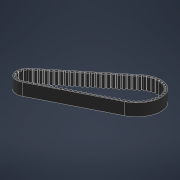
# Autodesk Inventor part: Parametric HTD Belt v1
Saved by Autodesk Inventor 2021 (Build 250183000, 183)
## iProperties
Created: 2020-06-05
Part Number: Parametric HTD Belt v1
Material: Rubber
Document SubType Name: Modeling
Designer: Bryce
Density: 0.93 g/cm^3
Appearance: Rubber - Black
Author: Bryce
Autodesk Inventor part; units mm, degrees
ref_plane "YZ Plane" through (0, 0, 0) normal (1, 0, 0) x (0, 1, 0)
ref_plane "XY Plane" through (0, 0, 0) normal (0, 0, 1) x (1, 0, 0)
sketch "top teeth placement" plane through (0, 0, 0) normal (0, 1, 0) x (-1, 0, 0)
  arc A0 (1.9259, -14.1939) -> (1.9259, 14.1939) centre (0, 0) ccw construction
  line L0 (1.9259, -14.1939) -> (-102.6854, -28.3878) construction
  line L1 (1.9259, 14.1939) -> (-102.6854, 28.3878) construction
  arc A1 (-102.6854, 28.3878) -> (-102.6854, -28.3878) centre (-106.5371, 0) ccw construction
  arc A2 (1.9259, -14.1939) -> (6.6643, -12.6792) centre (0, 0) ccw construction
  arc A3 (-107.1039, -28.6423) -> (-102.6854, -28.3878) centre (-106.5371, 0) ccw construction
  arc A4 (-112.0689, -28.1087) -> (-107.1039, -28.6423) centre (-106.5371, 0) ccw construction
  line L2 (1.9259, -14.1939) -> (0, 0) construction
  line L3 (0, 0) -> (6.6643, -12.6792) construction
  line L4 (-107.1039, -28.6423) -> (-106.5371, 0) construction
  line L5 (-106.5371, 0) -> (-112.0689, -28.1087) construction
  point P0 (-3.0287, -14.8661)
  point P1 (-7.9833, -15.5384)
  point P2 (-12.9379, -16.2106)
  point P3 (-17.8925, -16.8829)
  point P4 (-22.8471, -17.5551)
  point P5 (-27.8018, -18.2274)
  point P6 (-1.9025, 14.7133)
  point P7 (-6.8571, 15.3856)
  point P8 (-32.7564, -18.8996)
  point P9 (-37.711, -19.5719)
  point P10 (-42.6656, -20.2442)
  point P11 (-47.6202, -20.9164)
  point P12 (-52.5748, -21.5887)
  point P13 (-57.5294, -22.2609)
  point P14 (-62.484, -22.9332)
  point P15 (-67.4386, -23.6054)
  point P16 (-72.3932, -24.2777)
  point P17 (-77.3478, -24.9499)
  point P18 (-82.3024, -25.6222)
  point P19 (-87.257, -26.2944)
  point P20 (-92.2116, -26.9667)
  point P21 (-97.1662, -27.6389)
  point P22 (-102.1208, -28.3112)
  dimension "pitch" = 5
  dimension "r_d35" = 105
  dimension "r_d36" = 40
  dimension "d17" = 28.6479
  dimension "d18" = 57.2958
  dimension "d30" = 5
  dimension "d35" = 105.5697
  dimension "d36" = 41.1366
  dimension "d39" = 20
  dimension "d41" = 5
  dimension "d44" = 4.4303
  dimension "d45" = 97.7268
  dimension "d48" = 10
  dimension "d50" = 5
  dimension "d52" = 3.8634
  dimension "d62" = 5
  dimension "d71" = 106.5371
  constraints: 12 end point, 11 point on circle, 5 centre point, 4 coincident, 4 tangent, 3 concentric, 1 horizontal alignment, 1 point on line, 28 other
  measures "d17" diameter of A0
  measures "d18" diameter of A1
  measures "d30" distance of L2.start point (-3.029, -14.866)
  measures "d35" distance of L0.start L0.end
  measures "d52" distance of point (-1.902, 14.713) L1.start
  measures "d62" distance of point (-1.902, 14.713) point (-6.857, 15.386)
  measures "d71" distance of A1.centre point (0, 0)
sketch "htd profile" plane through (0, 0, 0) normal (0, 1, 0) x (-1, 0, 0)
  line L0 (-107.1039, -28.6423) -> (-106.5371, 0) construction
  arc A0 (-102.6854, 28.3878) -> (-102.6854, -28.3878) centre (-106.5371, 0) ccw construction
  arc A1 (3.2344, -12.9293) -> (0.3276, -13.3237) centre (1.7458, -12.8665) ccw
  line L1 (1.9259, -14.1939) -> (-102.6854, -28.3878) construction
  arc A2 (-0.0238, -13.8817) -> (0.3276, -13.3237) centre (-0.0816, -13.4556) ccw
  arc A3 (3.2344, -12.9293) -> (3.7219, -13.3735) centre (3.664, -12.9474) ccw
  line L2 (1.5454, -11.39) -> (1.8224, -13.4313) construction
  line L3 (4.3263, -13.2915) -> (3.7219, -13.3735)
  line L4 (-0.0238, -13.8817) -> (-0.6283, -13.9637)
  line L5 (4.4933, -14.5221) -> (-0.4613, -15.1943)
  line L6 (4.4933, -14.5221) -> (4.3263, -13.2915)
  line L7 (-0.4613, -15.1943) -> (-0.6283, -13.9637)
  line L8 (1.7458, -12.8665) -> (2.016, -14.8582) construction
  arc A4 (-105.6161, -27.5943) -> (-108.549, -27.5363) centre (-107.0774, -27.303) ccw
  arc A5 (-108.9822, -28.0335) -> (-108.549, -27.5363) centre (-108.9737, -27.6036) ccw
  arc A6 (-105.6161, -27.5943) -> (-105.2029, -28.1083) centre (-105.1944, -27.6784) ccw
  line L9 (-107.0479, -25.8133) -> (-107.0886, -27.8729) construction
  line L10 (-104.593, -28.1204) -> (-105.2029, -28.1083)
  line L11 (-108.9822, -28.0335) -> (-109.5921, -28.0214)
  line L12 (-104.6176, -29.362) -> (-109.6166, -29.2631)
  line L13 (-104.6176, -29.362) -> (-104.593, -28.1204)
  line L14 (-109.6166, -29.2631) -> (-109.5921, -28.0214)
  line L15 (-107.0774, -27.303) -> (-107.1171, -29.3126) construction
  line L16 (-104.6044, -28.6917) -> (-109.6034, -28.5928) construction
  line L17 (1.9259, 14.1939) -> (-102.6854, 28.3878) construction
  arc A7 (-3.5007, 13.8431) -> (-0.5939, 13.4487) centre (-2.0826, 13.3859) ccw
  arc A8 (-0.1065, 13.8929) -> (-0.5939, 13.4487) centre (-0.1643, 13.4668) ccw
  arc A9 (-3.5007, 13.8431) -> (-3.8522, 14.4011) centre (-3.91, 13.975) ccw
  line L18 (-2.2829, 11.9094) -> (-2.006, 13.9507) construction
  line L19 (-4.4566, 14.4831) -> (-3.8522, 14.4011)
  line L20 (-0.1065, 13.8929) -> (0.498, 13.8109)
  line L21 (-4.2896, 15.7138) -> (0.665, 15.0415)
  line L22 (-4.2896, 15.7138) -> (-4.4566, 14.4831)
  line L23 (0.665, 15.0415) -> (0.498, 13.8109)
  line L24 (-2.0826, 13.3859) -> (-1.8123, 15.3777) construction
  point P0 (0, 0)
  point P1 (-1.9025, 14.7133)
  dimension "d93" = 1.49
  dimension "d94" = 0.43
  dimension "d95" = 2.06
  dimension "d97" = 3.5
  dimension "d98" = 5
  dimension "d99" = 0.5715
  dimension "d101" = 3.78
  dimension "d102" = 1.49
  dimension "d103" = 0.43
  dimension "d104" = 2.06
  dimension "d105" = 3.5
  dimension "d106" = 5
  dimension "d107" = 3.78
  dimension "d109" = 0.5715
  dimension "d150" = 1.49
  dimension "d151" = 0.43
  dimension "d152" = 2.06
  dimension "d153" = 3.5
  dimension "d154" = 5
  dimension "d155" = 3.78
  dimension "d157" = 0.5715
  constraints: 44 end point, 21 point on circle, 19 tangent, 12 perpendicular, 9 centre point, 8 point on line, 7 parallel, 3 collinear, 3 equal radius, 3 midpoint, 1 line through centre
  measures "d93" radius of A1
  measures "d94" radius of A2
  measures "d95" distance of L2.start L2.end
  measures "d97" distance from line of L5 L2.start
  measures "d98" distance between parallel lines of L7 L6
  measures "d99" distance between parallel lines of L1 L4
  measures "d101" distance of L4.start L3.end
  measures "d102" radius of A4
  measures "d103" radius of A5
  measures "d104" distance of L9.start L9.end
  measures "d105" distance from line of L12 L9.start
  measures "d106" distance between parallel lines of L14 L13
  measures "d107" distance of L11.start L10.end
  measures "d109" distance between parallel lines of L16 L10
  measures "d150" radius of A7
  measures "d151" radius of A8
  measures "d152" distance of L18.start L18.end
  measures "d153" distance from line of L21 L18.start
  measures "d154" distance between parallel lines of L23 L22
  measures "d155" distance of L20.start L19.end
  measures "d157" distance between parallel lines of L17 L19
extrude "Top/Left Base Tooth" add sketch "htd profile" against normal mid plane 15 contours A3 L3 L6 L5 L7 L4 A2 A1
pattern_sketch "Top Teeth" of "Top/Left Base Tooth" from (-1.9259, 0, -14.1939) copies at (3.0287, 0, -14.8661) at (7.9833, 0, -15.5384) at (12.9379, 0, -16.2106) at (17.8925, 0, -16.8829) at (22.8471, 0, -17.5551) at (27.8018, 0, -18.2274) at (32.7564, 0, -18.8996) at (37.711, 0, -19.5719) at (42.6656, 0, -20.2442) at (47.6202, 0, -20.9164) at (52.5748, 0, -21.5887) at (57.5294, 0, -22.2609) at (62.484, 0, -22.9332) at (67.4386, 0, -23.6054) at (72.3932, 0, -24.2777) at (77.3478, 0, -24.9499) at (82.3024, 0, -25.6222) at (87.257, 0, -26.2944) at (92.2116, 0, -26.9667) at (97.1662, 0, -27.6389) at (102.1208, 0, -28.3112)
pattern_circular "Left Teeth" count 8 over 160 about axis through (0, 0, 0) along (0, 1, 0) of "Top/Left Base Tooth"
extrude "Right Base Tooth" add sketch "htd profile" along normal mid plane 15 contours A6 L10 L13 L12 L14 L11 A5 A4
pattern_circular "Right Teeth" count 19 over 180 about axis through (106.5371, 0, 0) along (0, -1, 0) of "Right Base Tooth"
sketch "bottom teeth placement" plane through (0, 0, 0) normal (0, 1, 0) x (-1, 0, 0)
  arc A0 (1.9259, -14.1939) -> (1.9259, 14.1939) centre (0, 0) ccw construction
  line L0 (1.9259, -14.1939) -> (-102.6854, -28.3878) construction
  line L1 (1.9259, 14.1939) -> (-102.6854, 28.3878) construction
  arc A1 (-102.6854, 28.3878) -> (-102.6854, -28.3878) centre (-106.5371, 0) ccw construction
  point P0 (-1.9025, 14.7133)
  point P1 (-6.8571, 15.3856)
  point P2 (-11.8117, 16.0578)
  point P3 (-16.7663, 16.7301)
  point P4 (-21.7209, 17.4023)
  point P5 (-26.6755, 18.0746)
  point P6 (-31.6301, 18.7468)
  point P7 (-36.5847, 19.4191)
  point P8 (-41.5393, 20.0913)
  point P9 (-46.4939, 20.7636)
  point P10 (-51.4485, 21.4358)
  point P11 (-56.4031, 22.1081)
  point P12 (-61.3577, 22.7803)
  point P13 (-66.3123, 23.4526)
  point P14 (-71.2669, 24.1248)
  point P15 (-76.2215, 24.7971)
  point P16 (-81.1761, 25.4694)
  point P17 (-86.1307, 26.1416)
  point P18 (-91.0853, 26.8139)
  point P19 (-96.0399, 27.4861)
  point P20 (-100.9945, 28.1584)
  dimension "d144" = 5
  dimension "d147" = 40
  dimension "pitch" = 5
  dimension "d123" = 28.6479
  dimension "d124" = 57.2958
  dimension "d126" = 105.5697
  dimension "d127" = 41.1366
  dimension "d131" = 97.7268
  dimension "d134" = 3.8634
  dimension "d135" = 5
  dimension "d136" = 106.5371
  constraints: 4 end point, 4 point on circle, 4 tangent, 2 centre point, 2 coincident, 1 horizontal alignment, 1 point on line, 21 other
  measures "d123" diameter of A0
  measures "d124" diameter of A1
  measures "d126" distance of L0.start L0.end
  measures "d134" distance of point (-1.902, 14.713) L1.start
  measures "d135" distance of point (-1.902, 14.713) point (-6.857, 15.386)
  measures "d136" distance of A1.centre point (0, 0)
extrude "Bottom Base Tooth" add sketch "htd profile" along normal mid plane 15 contours A9 L19 L22 L21 L23 L20 A8 A7
pattern_sketch "Bottom Teeth" of "Bottom Base Tooth" from (1.9025, 0, 14.7133) copies at (6.8571, 0, 15.3856) at (11.8117, 0, 16.0578) at (16.7663, 0, 16.7301) at (21.7209, 0, 17.4023) at (26.6755, 0, 18.0746) at (31.6301, 0, 18.7468) at (36.5847, 0, 19.4191) at (41.5393, 0, 20.0913) at (46.4939, 0, 20.7636) at (51.4485, 0, 21.4358) at (56.4031, 0, 22.1081) at (61.3577, 0, 22.7803) at (66.3123, 0, 23.4526) at (71.2669, 0, 24.1248) at (76.2215, 0, 24.7971) at (81.1761, 0, 25.4694) at (86.1307, 0, 26.1416) at (91.0853, 0, 26.8139) at (96.0399, 0, 27.4861) at (100.9945, 0, 28.1584)
sketch "Sketch7" plane through (0, 0, 0) normal (0, 1, 0) x (-1, 0, 0)
  line L0 (1.9259, 14.1939) -> (-102.6854, 28.3878) construction
  arc A0 (1.9259, -14.1939) -> (1.9259, 14.1939) centre (0, 0) ccw construction
  line L1 (1.9259, -14.1939) -> (-102.6854, -28.3878) construction
  arc A1 (-102.6854, 28.3878) -> (-102.6854, -28.3878) centre (-106.5371, 0) ccw construction
  line L2 (1.849, 13.6276) -> (-102.7622, 27.8215)
  arc A2 (-102.7622, 27.8215) -> (-102.7622, -27.8215) centre (-106.5371, 0) ccw
  line L3 (-102.7622, -27.8215) -> (1.849, -13.6276)
  arc A3 (1.849, -13.6276) -> (1.849, 13.6276) centre (0, 0) ccw
  line L4 (-102.5549, -29.3494) -> (2.0563, -15.1555)
  arc A4 (2.0563, -15.1555) -> (2.0563, 15.1555) centre (0, 0) ccw
  line L5 (2.0563, 15.1555) -> (-102.5549, 29.3494)
  arc A5 (-102.5549, 29.3494) -> (-102.5549, -29.3494) centre (-106.5371, 0) ccw
  line L6 (-0.0238, -13.8817) -> (-1.2327, -14.0457) construction
  line L7 (-104.5079, -29.3116) -> (4.4933, -14.5221) construction
  arc A6 (3.2344, -12.9293) -> (0.3276, -13.3237) centre (1.7458, -12.8665) ccw construction
  arc A7 (3.2344, -12.9293) -> (0.3276, -13.3237) centre (1.7458, -12.8665) ccw construction
  line L8 (1.5454, -11.39) -> (1.849, -13.6276) construction
  dimension "d163" = 3.8
  constraints: 10 end point, 9 point on circle, 4 centre point, 2 point on line, 1 coincident, 1 collinear, 1 perpendicular, 6 other
  measures "d163" distance from line of L4 point (1.545, -11.39)
extrude "Belt" add sketch "Sketch7" along normal mid plane 15
equation "\"pitch\" = 5"
equation "\"r_d36\" = 40"
equation "\"d30\" = pitch"
equation "\"d41\" = pitch"
equation "\"d44\" = pitch + r_d35 - d35"
equation "\"d50\" = pitch"
equation "\"d62\" = pitch"
equation "\"d144\" = 5"
equation "\"d147\" = 40"
equation "\"r_d45\" = 95"
equation "\"pulley_1_angle\" = 20deg"
equation "\"pulley_2_angle\" = 10deg"
equation "\"d108\" = 5"
equation "\"d156\" = 5"
equation "\"center_distance\" = 106.53707"
equation "\"f_d35\" = 105"
equation "\"htd_pld\" = 0.5715"
equation "\"missing_tooth_bottom_right_round\" = 0"
equation "\"missing_tooth_bottom_right_straight\" = 0"
equation "\"missing_tooth_bottom_left\" = 0"
equation "\"belt_width\" = 15"
body "Solid3"
